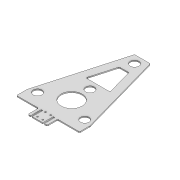
# Autodesk Inventor part: Foam_wing_mount_clamp
Saved by Autodesk Inventor 2022 (Build 260153000, 153)
## iProperties
Created: 2022-06-29
Part Number: Foam_wing_mount_clamp
Material: Generic
Document SubType Name: Modeling
Designer: dell
Density: 1 g/cm^3
Appearance: Default
Mass: 22.4639 g
Surface Area: 248.081 cm^2
Volume: 22.4639 cm^3
Author: dell
Autodesk Inventor part; units mm, degrees
ref_plane "YZ Plane" through (0, 0, 0) normal (1, 0, 0) x (0, 1, 0)
ref_plane "XZ Plane" through (0, 0, 0) normal (0, 1, 0) x (-1, 0, 0)
ref_plane "XY Plane" through (0, 0, 0) normal (0, 0, 1) x (1, 0, 0)
sketch "Sketch1" plane through (0, 0, 0) normal (0, 1, 0) x (-1, 0, 0)
  line L0 (0, 0) -> (20, 0)
  line L1 (20, 0) -> (20, -20)
  line L2 (20, -20) -> (0, -20)
  line L3 (0, -20) -> (0, 0)
  line L4 (70, -20) -> (-50, -20)
  line L5 (-50, -20) -> (-50, -40)
  line L6 (-50, -40) -> (70, -40)
  line L7 (70, -40) -> (70, -20)
  line L8 (10, 0) -> (10, -20) construction
  line L9 (70, -40) -> (25, -200)
  line L10 (25, -200) -> (-5, -200)
  line L11 (-5, -200) -> (-50, -40)
  circle A0 centre (55, -45) radius 8.25
  circle A1 centre (-35, -45) radius 8.25
  circle A2 centre (10, -185) radius 8.25
  circle A3 centre (10, -100) radius 8.25
  circle A4 centre (15, -5) radius 1.5
  circle A5 centre (15, -20) radius 1.5
  circle A6 centre (5, -5) radius 1.5
  circle A7 centre (5, -20) radius 1.5
  line L12 (28.1, -20) -> (23.1, -20)
  line L13 (23.1, -20) -> (23.1, 0)
  line L14 (23.1, 0) -> (28.1, 0)
  line L15 (28.1, 0) -> (28.1, -20)
  line L16 (-8.1, -20) -> (-3.1, -20)
  line L17 (-3.1, -20) -> (-3.1, 0)
  line L18 (-3.1, 0) -> (-8.1, 0)
  line L19 (-8.1, 0) -> (-8.1, -20)
  line L20 (33.3243, -115) -> (-13.3243, -115)
  line L21 (-13.3243, -115) -> (0.7382, -165)
  line L22 (0.7382, -165) -> (19.2618, -165)
  line L23 (19.2618, -165) -> (33.3243, -115)
  circle A8 centre (10, -65) radius 20
  point P0 (10, -10)
  point P1 (20, -20)
  point P2 (0, -20)
  point P3 (-3.1, -20)
  point P4 (23.1, -20)
  point P5 (10, -40)
  point P6 (-5, -40)
  dimension "d0" = 20
  dimension "d1" = 20
  dimension "d2" = 120
  dimension "d3" = 60
  dimension "d4" = 20
  dimension "d6" = 200
  dimension "d7" = 45
  dimension "d8" = 45
  dimension "d9" = 16.5
  dimension "d10" = 16.5
  dimension "d11" = 16.5
  dimension "d12" = 16.5
  dimension "d13" = 15
  dimension "d14" = 15
  dimension "d15" = 25
  dimension "d16" = 25
  dimension "d17" = 15
  dimension "d18" = 100
  dimension "d23" = 3
  dimension "d24" = 3
  dimension "d25" = 3
  dimension "d26" = 3
  dimension "d27" = 5
  dimension "d28" = 5
  dimension "d29" = 5
  dimension "d30" = 5
  dimension "d31" = 0
  dimension "d32" = 0
  dimension "d33" = 5
  dimension "d34" = 5
  dimension "d38" = 3.1
  dimension "d39" = 3.1
  dimension "d40" = 5
  dimension "d41" = 5
  dimension "d56" = 15
  dimension "d57" = 15
  dimension "d58" = 20
  dimension "d59" = 15
  dimension "d64" = 40
  dimension "d66" = 35
  constraints: 48 end point, 11 parallel, 9 centre point, 6 horizontal, 5 perpendicular, 4 point on line, 3 midpoint, 2 vertical alignment, 1 collinear
  measures "d0" distance of L2.end L0.start
  measures "d1" distance of L0.start L0.end
  measures "d2" distance of L5.end L6.end
  measures "d3" distance between parallel lines of L8 L5
  measures "d4" distance of L4.end L5.end
  measures "d6" distance between parallel lines of L0 L10
  measures "d7" horizontal distance of L5.end L10.end
  measures "d8" distance from line of L7 L9.end
  measures "d9" diameter of A0
  measures "d10" diameter of A1
  measures "d11" diameter of A2
  measures "d12" diameter of A3
  measures "d13" distance from line of L7 A0.centre
  measures "d14" distance from line of L5 A1.centre
  measures "d15" distance from line of L4 A1.centre
  measures "d16" distance from line of L4 A0.centre
  measures "d17" distance from line of L10 A2.centre
  measures "d18" distance from line of L10 A3.centre
  measures "d23" diameter of A4
  measures "d24" diameter of A5
  measures "d25" diameter of A6
  measures "d26" diameter of A7
  measures "d27" distance from line of L3 A6.centre
  measures "d28" distance from line of L1 A4.centre
  measures "d29" distance from line of L1 A5.centre
  measures "d30" distance from line of L3 A7.centre
  measures "d31" distance from line of L4 A7.centre
  measures "d32" distance from line of L4 A5.centre
  measures "d33" distance from line of L0 A4.centre
  measures "d34" distance from line of L0 A6.centre
  measures "d38" distance between parallel lines of L3 L17
  measures "d39" distance between parallel lines of L1 L13
  measures "d40" distance of L17.end L18.end
  measures "d41" distance of L13.end L14.end
  measures "d56" distance between parallel lines of L11 L21
  measures "d57" distance between parallel lines of L9 L23
  measures "d58" distance from line of A2.centre L22
  measures "d59" distance from line of A3.centre L20
  measures "d64" diameter of A8
  measures "d66" distance of A3.centre A8.centre
extrude "Extrusion1" add sketch "Sketch1" along normal blind 2 contours L0 L1 L2 A5 A7 L3 | L2 A7 A5 L4 L7 L6 A0 A1 L5 | L4 L19 L18 L17 | L13 L14 L15 L4 | L6 A1 A0 L9 L10 L11
fillet "Fillet1" radius 2 14 edges at (-70, 1, -20) (50, 1, -20) (-25, 1, -200) (5, 1, -200) (-28.1, 1, 0) (8.1, 1, 0) (-28.1, 1, -20) (8.1, 1, -20) (50, 1, -40) (-70, 1, -40) (-33.3243, 1, -115) (13.3243, 1, -115) (-0.7382, 1, -165) (-19.2618, 1, -165)
sketch "Sketch6" plane through (0, 2, 0) normal (0, 1, 0) x (1, 0, 0)
  arc A0 (-69.9253, 40.2656) -> (-70, 39.7241) centre (-68, 39.7241) ccw projected
  line L0 (-70, 39.7241) -> (-70, 22) projected
  arc A1 (-70, 22) -> (-68, 20) centre (-68, 22) ccw projected
  line L1 (-68, 20) -> (-30.1, 20) projected
  arc A2 (-28.1, 18) -> (-30.1, 20) centre (-30.1, 18) ccw projected
  line L2 (-28.1, 18) -> (-28.1, 2) projected
  arc A3 (-28.1, 2) -> (-26.1, 0) centre (-26.1, 2) ccw projected
  line L3 (-26.1, 0) -> (-23.1, 0) projected
  line L4 (-23.1, 0) -> (-23.1, 20) projected
  line L5 (-23.1, 20) -> (-20, 20) projected
  line L6 (-20, 20) -> (-20, 0) projected
  line L7 (-20, 0) -> (0, 0) projected
  line L8 (0, 0) -> (0, 20) projected
  line L9 (0, 20) -> (3.1, 20) projected
  line L10 (3.1, 20) -> (3.1, 0) projected
  line L11 (3.1, 0) -> (6.1, 0) projected
  arc A4 (6.1, 0) -> (8.1, 2) centre (6.1, 2) ccw projected
  line L12 (8.1, 2) -> (8.1, 18) projected
  arc A5 (10.1, 20) -> (8.1, 18) centre (10.1, 18) ccw projected
  line L13 (10.1, 20) -> (48, 20) projected
  arc A6 (48, 20) -> (50, 22) centre (48, 22) ccw projected
  line L14 (50, 22) -> (50, 39.7241) projected
  arc A7 (50, 39.7241) -> (49.9253, 40.2656) centre (48, 39.7241) ccw projected
  line L15 (49.9253, 40.2656) -> (5.4102, 198.5415) projected
  arc A8 (5.4102, 198.5415) -> (3.4849, 200) centre (3.4849, 198) ccw projected
  line L16 (3.4849, 200) -> (-23.4849, 200) projected
  arc A9 (-23.4849, 200) -> (-25.4102, 198.5415) centre (-23.4849, 198) ccw projected
  line L17 (-25.4102, 198.5415) -> (-69.9253, 40.2656) projected
  circle A10 centre (-5, 20) radius 1.5 projected
  circle A11 centre (-5, 5) radius 1.5 projected
  circle A12 centre (-15, 5) radius 1.5 projected
  circle A13 centre (-15, 20) radius 1.5 projected
  circle A14 centre (35, 45) radius 8.25 projected
  circle A15 centre (-10, 65) radius 20 projected
  circle A16 centre (-55, 45) radius 8.25 projected
  circle A17 centre (-10, 185) radius 8.25 projected
  circle A18 centre (-10, 100) radius 8.25 projected
  line L18 (-32.6095, 117.5415) -> (-19.672, 163.5415) projected
  arc A19 (-17.7467, 165) -> (-19.672, 163.5415) centre (-17.7467, 163) ccw projected
  line L19 (-17.7467, 165) -> (-2.2533, 165) projected
  arc A20 (-0.328, 163.5415) -> (-2.2533, 165) centre (-2.2533, 163) ccw projected
  line L20 (-0.328, 163.5415) -> (12.6095, 117.5415) projected
  arc A21 (10.6842, 115) -> (12.6095, 117.5415) centre (10.6842, 117) ccw projected
  line L21 (10.6842, 115) -> (-30.6842, 115) projected
  arc A22 (-32.6095, 117.5415) -> (-30.6842, 115) centre (-30.6842, 117) ccw projected
  dimension "d67" = 16.2
  dimension "d68" = 16.2
  dimension "d69" = 16.2
  dimension "d70" = 16.2
  dimension "d71" = 3
  dimension "d72" = 3
  dimension "d73" = 3
  dimension "d74" = 3
  constraints: 8 centre point, 4 coincident
sketch "Sketch8" plane through (0, 2, 0) normal (0, 1, 0) x (1, 0, 0)
  circle A0 centre (-10, 185) radius 11.25 projected
  circle A1 centre (-10, 100) radius 11.25 projected
  circle A2 centre (35, 45) radius 11.25 projected
  circle A3 centre (-55, 45) radius 11.25 projected
  arc A4 (-69.9253, 40.2656) -> (-70, 39.7241) centre (-68, 39.7241) ccw projected
  line L0 (-70, 39.7241) -> (-70, 22) projected
  arc A5 (-70, 22) -> (-68, 20) centre (-68, 22) ccw projected
  line L1 (-68, 20) -> (-30.1, 20) projected
  arc A6 (-28.1, 18) -> (-30.1, 20) centre (-30.1, 18) ccw projected
  line L2 (-28.1, 18) -> (-28.1, 2) projected
  arc A7 (-28.1, 2) -> (-26.1, 0) centre (-26.1, 2) ccw projected
  line L3 (-26.1, 0) -> (-23.1, 0) projected
  line L4 (-23.1, 0) -> (-23.1, 20) projected
  line L5 (-23.1, 20) -> (-20, 20) projected
  line L6 (-20, 20) -> (-20, 0) projected
  line L7 (-20, 0) -> (0, 0) projected
  line L8 (0, 0) -> (0, 20) projected
  line L9 (0, 20) -> (3.1, 20) projected
  line L10 (3.1, 20) -> (3.1, 0) projected
  line L11 (3.1, 0) -> (6.1, 0) projected
  arc A8 (6.1, 0) -> (8.1, 2) centre (6.1, 2) ccw projected
  line L12 (8.1, 2) -> (8.1, 18) projected
  arc A9 (10.1, 20) -> (8.1, 18) centre (10.1, 18) ccw projected
  line L13 (10.1, 20) -> (48, 20) projected
  arc A10 (48, 20) -> (50, 22) centre (48, 22) ccw projected
  line L14 (50, 22) -> (50, 39.7241) projected
  arc A11 (50, 39.7241) -> (49.9253, 40.2656) centre (48, 39.7241) ccw projected
  line L15 (49.9253, 40.2656) -> (5.4102, 198.5415) projected
  arc A12 (5.4102, 198.5415) -> (3.4849, 200) centre (3.4849, 198) ccw projected
  line L16 (3.4849, 200) -> (-23.4849, 200) projected
  arc A13 (-23.4849, 200) -> (-25.4102, 198.5415) centre (-23.4849, 198) ccw projected
  line L17 (-25.4102, 198.5415) -> (-69.9253, 40.2656) projected
  circle A14 centre (-5, 20) radius 1.5 projected
  circle A15 centre (-5, 5) radius 1.5 projected
  circle A16 centre (-15, 5) radius 1.5 projected
  circle A17 centre (-15, 20) radius 1.5 projected
  circle A18 centre (-10, 65) radius 20 projected
  line L18 (-32.6095, 117.5415) -> (-19.672, 163.5415) projected
  arc A19 (-17.7467, 165) -> (-19.672, 163.5415) centre (-17.7467, 163) ccw projected
  line L19 (-17.7467, 165) -> (-2.2533, 165) projected
  arc A20 (-0.328, 163.5415) -> (-2.2533, 165) centre (-2.2533, 163) ccw projected
  line L20 (-0.328, 163.5415) -> (12.6095, 117.5415) projected
  arc A21 (10.6842, 115) -> (12.6095, 117.5415) centre (10.6842, 117) ccw projected
  line L21 (10.6842, 115) -> (-30.6842, 115) projected
  arc A22 (-32.6095, 117.5415) -> (-30.6842, 115) centre (-30.6842, 117) ccw projected
  circle A23 centre (-15, 5) radius 1.6
  circle A24 centre (-15, 20) radius 1.6
  circle A25 centre (-5, 20) radius 1.6
  circle A26 centre (-5, 5) radius 1.6
  dimension "d79" = 0.1
  dimension "d80" = 0.1
  dimension "d81" = 0.1
  dimension "d82" = 0.1
  constraints: 4 centre point
  measures "d79" radial gap between concentric circles of A16 A23
  measures "d80" radial gap between concentric circles of A17 A24
  measures "d81" radial gap between concentric circles of A14 A25
  measures "d82" radial gap between concentric circles of A15 A26
equation "\"d3\" = 0.5 * d2"
body "Solid1"
